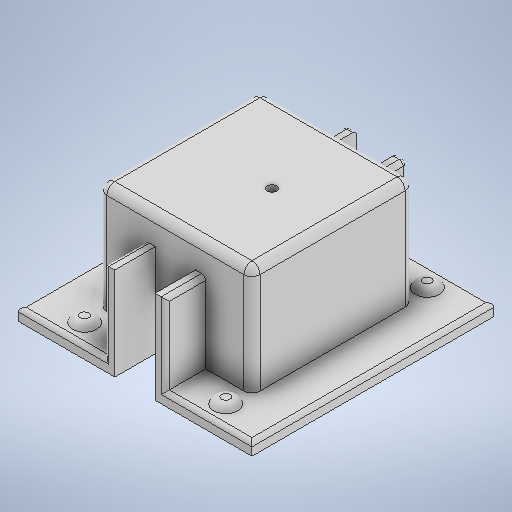
# Autodesk Inventor part: liquid_port_v07_IRBEAMS_v11
Saved by Autodesk Inventor 2025.2 (Build 292293000, 293)
## iProperties
Created: 2021-04-13
Part Number: liquid_port_v07_IRBEAMS_v11
Material: Generic
Document SubType Name: Modeling
Designer: KAMPFF-LAB-BEHAVIOR
Density: 1 g/cm^3
Appearance: Default
Author: KAMPFF-LAB-BEHAVIOR
Autodesk Inventor part; units mm, degrees
ref_plane "YZ Plane" through (0, 0, 0) normal (1, 0, 0) x (0, 1, 0)
ref_plane "XZ Plane" through (0, 0, 0) normal (0, 1, 0) x (-1, 0, 0)
ref_plane "XY Plane" through (0, 0, 0) normal (0, 0, 1) x (1, 0, 0)
ref_plane "Work Plane5" through (0, 3, 0) normal (0, 1, 0) x (1, 0, 0)
sketch "Sketch45" plane through (0, 3, 0) normal (0, 1, 0) x (1, 0, 0)
  line L0 (35, -20) -> (-3, -20)
  line L1 (-3, -20) -> (-3, 20)
  line L2 (-3, 20) -> (35, 20)
  line L3 (35, 20) -> (35, -20)
  point P0 (0, 0)
  dimension "d142" = 38
  dimension "d143" = 40
  constraints: 8 end point, 2 parallel, 1 horizontal, 1 perpendicular
  measures "d142" distance of L1.end L2.end
  measures "d143" distance of L0.end L1.end
extrude "Extrusion34" add sketch "Sketch45" along normal blind 30
ref_plane "Work Plane2" through (0, 0, 0) normal (0, -1, 0) x (1, 0, 0)
sketch "Sketch47" plane through (0, 0, 0) normal (0, -1, 0) x (1, 0, 0)
  circle A0 centre (16, 0) radius 18
  point P0 (0, 0)
  dimension "d146" = 36
  constraints: 1 centre point
  measures "d146" diameter of A0
extrude "Extrusion35" cut sketch "Sketch47" against normal blind 30 draft -15
ref_plane "Work Plane1" through (0, 3, 0) normal (0, 1, 0) x (1, 0, 0)
sketch "Sketch74" plane through (0, 33, 0) normal (0, 1, 0) x (1, 0, 0)
  circle A0 centre (20, 0) radius 1.15
  point P0 (0, 0)
  dimension "d210" = 2.3
  constraints: 1 centre point
  measures "d210" diameter of A0
extrude "Extrusion51" cut sketch "Sketch74" against normal blind 10
sketch "Sketch77" plane through (0, 3, 0) normal (0, -1, 0) x (1, 0, 0)
  circle A0 centre (16, 0) radius 17.5
  point P0 (0, 0)
  dimension "d219" = 35
  constraints: 1 centre point
  measures "d219" diameter of A0
sketch "Sketch78" plane through (0, 3, 0) normal (0, -1, 0) x (1, 0, 0)
  line L0 (45, -30) -> (-13, -30)
  line L1 (-13, -30) -> (-13, 30)
  line L2 (-13, 30) -> (45, 30)
  line L3 (45, 30) -> (45, -30)
  line L4 (45, -30) -> (-13, 30) construction
  line L5 (-13, -30) -> (45, 30) construction
  point P0 (0, 0)
  point P1 (16, 0)
  dimension "d220" = 58
  dimension "d221" = 60
  constraints: 12 end point, 2 midpoint, 2 parallel, 1 horizontal, 1 perpendicular
  measures "d220" distance of L1.end L2.end
  measures "d221" distance of L0.end L1.end
extrude "Extrusion53" add sketch "Sketch78" against normal blind 3
extrude "Extrusion54" cut sketch "Sketch77" against normal blind 3
sketch "Sketch81" plane through (0, 3, 0) normal (0, -1, 0) x (1, 0, 0)
  circle A0 centre (33.5, -25) radius 2.7
  line L0 (-13, -30) -> (45, -30)
  line L1 (45, -30) -> (45, 30) projected
  circle A1 centre (-1.5, -25) radius 2.7
  circle A2 centre (-1.5, 25) radius 2.7
  circle A3 centre (33.5, 25) radius 2.7
  point P0 (0, 0)
  dimension "mag_D" = 5.4
  dimension "d232" = 5
  dimension "d233" = 11.5
  dimension "d236" = 5.4
  dimension "d243" = 5.4
  dimension "d247" = 5.4
  constraints: 4 centre point, 2 end point
  measures "mag_D" diameter of A0
  measures "d232" distance from line of A0.centre L0
  measures "d233" distance from line of L1 A0.centre
  measures "d236" diameter of A1
  measures "d243" diameter of A2
  measures "d247" diameter of A3
extrude "Extrusion56" cut sketch "Sketch81" against normal blind 30
sketch "Sketch85" plane through (0, 6, 0) normal (0, 1, 0) x (1, 0, 0)
  circle A0 centre (-1.5, -25) radius 2.7 projected
  circle A1 centre (33.5, -25) radius 2.7 projected
  circle A2 centre (-1.5, 25) radius 2.7 projected
  circle A3 centre (33.5, 25) radius 2.7 projected
  line L0 (23.5, -30) -> (8.5, -30)
  line L1 (8.5, -30) -> (8.5, -20)
  line L2 (8.5, -20) -> (23.5, -20)
  line L3 (23.5, -20) -> (23.5, -30)
  line L4 (23.5, -30) -> (8.5, -20) construction
  line L5 (8.5, -30) -> (23.5, -20) construction
  line L6 (23.5, 30) -> (8.5, 30)
  line L7 (8.5, 30) -> (8.5, 20)
  line L8 (8.5, 20) -> (23.5, 20)
  line L9 (23.5, 20) -> (23.5, 30)
  line L10 (23.5, 30) -> (8.5, 20) construction
  line L11 (8.5, 30) -> (23.5, 20) construction
  point P0 (0, 0)
  point P1 (16, -25)
  point P2 (16, 25)
  dimension "d256" = 15
  dimension "d257" = 10
  dimension "d258" = 15
  dimension "d287" = 12.5
  dimension "d288" = 12.5
  constraints: 24 end point, 4 midpoint, 4 parallel, 2 horizontal, 2 perpendicular
  measures "d256" distance of L1.end L2.end
  measures "d257" distance of L0.end L1.end
  measures "d258" distance of L8.end L7.end
extrude "Extrusion58" add sketch "Sketch85" along normal blind 20 contours L0 L1 L2 L3 | L9 L8 L7 L6
sketch "Sketch86" plane through (0, 26, 0) normal (0, 1, 0) x (1, 0, 0)
  line L0 (11, 20) -> (21, 20)
  line L1 (21, 20) -> (21, 30)
  line L2 (21, 30) -> (11, 30)
  line L3 (11, 30) -> (11, 20)
  line L4 (23.5, 20) -> (8.5, 20) projected
  line L5 (8.5, -30) -> (23.5, -30) projected
  line L6 (11, -30) -> (21, -30)
  line L7 (21, -30) -> (21, -20)
  line L8 (21, -20) -> (11, -20)
  line L9 (11, -20) -> (11, -30)
  line L10 (8.5, 30) -> (8.5, 20) projected
  line L11 (8.5, -20) -> (8.5, -30) projected
  point P0 (0, 0)
  point P1 (11, -25)
  dimension "d261" = 10
  dimension "d262" = 10
  dimension "d263" = 10
  dimension "d264" = 10
  dimension "d265" = 2.5
  dimension "d266" = 2.5
  constraints: 16 end point, 4 parallel, 2 horizontal, 2 perpendicular, 1 collinear, 1 midpoint, 1 point on line
  measures "d261" distance of L2.end L1.end
  measures "d262" distance of L1.end L0.end
  measures "d263" distance of L8.end L7.end
  measures "d264" distance of L7.end L6.end
  measures "d265" distance between parallel lines of L3 L10
  measures "d266" distance from line of point (11, -25) L11
extrude "Extrusion59" cut sketch "Sketch86" against normal blind 23.5
sketch "Sketch87" plane through (35, 33, -20) normal (0, 0, -1) x (-1, 0, 0)
  line L0 (24, -30) -> (14, -30) projected
  circle A0 centre (19, -25.9) radius 2.1
  point P0 (35, -33)
  point P1 (19, -30)
  dimension "d269" = 4.2
  dimension "d270" = 4.1
  constraints: 1 centre point, 1 midpoint
  measures "d269" diameter of A0
  measures "d270" distance of point (19, -30) A0.centre
extrude "Extrusion60" cut sketch "Sketch87" against normal blind 40.25
sketch "Sketch88" plane through (35, 33, -20) normal (0, 0, -1) x (-1, 0, 0)
  circle A0 centre (19, -25.9) radius 2.1 projected
  circle A1 centre (19, -25.9) radius 4
  point P0 (35, -33)
  dimension "d273" = 8
  constraints: 1 centre point, 1 coincident
  measures "d273" diameter of A1
extrude "Extrusion61" cut sketch "Sketch88" against normal blind 1.5
sketch "Sketch89" plane through (-3, 33, 20) normal (0, 0, 1) x (1, 0, 0)
  circle A0 centre (19, -25.9) radius 2.1 projected
  circle A1 centre (19, -25.9) radius 4
  point P0 (3, -33)
  dimension "d276" = 8
  constraints: 1 centre point, 1 coincident
  measures "d276" diameter of A1
extrude "Extrusion62" cut sketch "Sketch89" against normal blind 1.5
sketch "Sketch90" plane through (-3, 33, 20) normal (0, 0, 1) x (1, 0, 0)
  circle A0 centre (19, -25.9) radius 2.1 projected
  line L0 (19, -25.9) -> (19, -15.9) construction
  circle A1 centre (19, -15.9) radius 2.25
  point P0 (3, -33)
  dimension "d279" = 10
  dimension "d280" = 4.5
  constraints: 2 end point, 1 centre point, 1 coincident, 1 vertical
  measures "d279" distance of L0.start L0.end
  measures "d280" diameter of A1
extrude "Extrusion63" cut sketch "Sketch90" against normal blind 5.7 contours A1
sketch "Sketch91" plane through (35, 33, -20) normal (0, 0, -1) x (-1, 0, 0)
  circle A0 centre (19, -25.9) radius 2.1 projected
  line L0 (19, -25.9) -> (19, -15.9) construction
  circle A1 centre (19, -15.9) radius 2.25
  point P0 (35, -33)
  dimension "d283" = 10
  dimension "d284" = 4.5
  constraints: 2 end point, 1 centre point, 1 coincident, 1 vertical
  measures "d283" distance of L0.start L0.end
  measures "d284" diameter of A1
extrude "Extrusion64" cut sketch "Sketch91" against normal blind 5.7 contours A1
fillet "Fillet1" radius 1 16 edges at (45, 6, 0) (34.25, 6, 30) (23.5, 16, 30) (23.5, 26, 25) (23.5, 16, -30) (23.5, 26, -25) (34.25, 6, -30) (-2.25, 6, -30) (8.5, 16, -30) (9.75, 26, -30) (22.25, 26, -30) (8.5, 26, -25) (-13, 6, 0) (-2.25, 6, 30) (8.5, 16, 30) (8.5, 26, 25)
fillet "Fillet2" radius 2 8 edges at (35, 19.5, -20) (16, 33, -20) (-3, 19.5, -20) (-3, 33, 0) (16, 33, 20) (35, 33, 0) (35, 19.5, 20) (-3, 19.5, 20)
sketch "Sketch92" plane through (0, 6, 0) normal (0, 1, 0) x (1, 0, 0)
  circle A0 centre (-1.5, -25) radius 2.7 projected
  circle A1 centre (-1.5, 25) radius 2.7 projected
  circle A2 centre (33.5, 25) radius 2.7 projected
  circle A3 centre (33.5, -25) radius 2.7 projected
  circle A4 centre (-1.5, -25) radius 3
  circle A5 centre (-1.5, 25) radius 3
  circle A6 centre (33.5, 25) radius 3
  circle A7 centre (33.5, -25) radius 3
  point P0 (0, 0)
  dimension "d291" = 6
  dimension "d292" = 6
  dimension "d293" = 6
  dimension "d294" = 6
  constraints: 4 centre point, 4 coincident
  measures "d291" diameter of A4
  measures "d292" diameter of A5
  measures "d293" diameter of A6
  measures "d294" diameter of A7
extrude "Extrusion65" add sketch "Sketch92" along normal blind 1.5 contours A0 | A1 | A2 | A3 | A4 | A5 | A6 | A7
fillet "Fillet3" radius 2 4 edges at (-4.5, 7.5, -25) (30.5, 7.5, -25) (-4.5, 7.5, 25) (30.5, 7.5, 25)
equation "\"d236\" = mag_D"
equation "\"d243\" = mag_D"
equation "\"d247\" = mag_D"
equation "\"ScrewDiameter\" = 4.5"
equation "\"LEDOuterDiameter\" = 8"
equation "\"LEDInnerDiameter\" = 4.2"
equation "\"SensorHeight\" = 12.5"
equation "\"EdgeDistance\" = 4.1"
body "Solid9"
